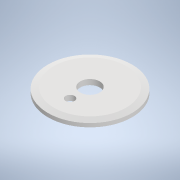
# Autodesk Inventor part: top_flange
Saved by Autodesk Inventor 2021 (Build 250183000, 183)
## iProperties
Created: 2024-01-29
Part Number: top_flange
Material: Generic
Document SubType Name: Modeling
Designer: Sebastián
Density: 1 g/cm^3
Appearance: Default
Author: Sebastián
Autodesk Inventor part; units mm, degrees
ref_plane "YZ Plane" through (0, 0, 0) normal (1, 0, 0) x (0, 1, 0)
ref_plane "XZ Plane" through (0, 0, 0) normal (0, 1, 0) x (-1, 0, 0)
ref_plane "XY Plane" through (0, 0, 0) normal (0, 0, 1) x (1, 0, 0)
sketch "Sketch1" plane through (0, 0, 0) normal (1, 0, 0) x (0, 1, 0)
  line L0 (0, 95) -> (8.4, 95)
  line L1 (8.4, 95) -> (12, 81.5646)
  line L2 (12, 81.5646) -> (12, 0)
  line L3 (12, 0) -> (0, 0)
  line L4 (0, 0) -> (0, 73.5)
  line L5 (0, 73.5) -> (3.5, 73.5)
  line L6 (3.5, 73.5) -> (3.5, 76.5)
  line L7 (3.5, 76.5) -> (0, 76.5)
  line L8 (0, 76.5) -> (0, 95)
  line L9 (0, 114) -> (0, -19) construction
  line L10 (-2.4, 0) -> (14.4, 0) projected
  dimension "d0" = 95
  dimension "d1" = 12
  dimension "d2" = 8.4
  dimension "d3" = 3.5
  dimension "d4" = 3
  dimension "d5" = 73.5
  dimension "d6" = 165
  constraints: 19 end point, 6 perpendicular, 3 point on line, 1 horizontal
  measures "d0" distance of L3.end L0.start
  measures "d1" distance of L3.end L2.end
  measures "d2" distance of L0.start L0.end
  measures "d3" distance of L4.end L5.end
  measures "d4" distance of L5.end L6.end
  measures "d5" distance of L3.end L4.end
  measures "d6" angle of L2 L1
revolve "Revolution1" add sketch "Sketch1" angle 360 about axis through (0, -10, 0) along (0, 1, 0)
sketch "Sketch2" plane through (0, 0, 0) normal (0, -1, 0) x (1, 0, 0)
  circle A0 centre (0, 0) radius 81.5646 projected
  circle A1 centre (0, 0) radius 22
  circle A2 centre (0, 60) radius 10
  dimension "d8" = 44
  dimension "d9" = 20
  dimension "d10" = 60
  constraints: 2 centre point, 1 coincident
  measures "d8" diameter of A1
  measures "d9" diameter of A2
  measures "d10" distance of point (0, 0) A2.centre
extrude "Extrusion1" cut sketch "Sketch2" against normal through all contours A1 | A2
body "Solid1"
